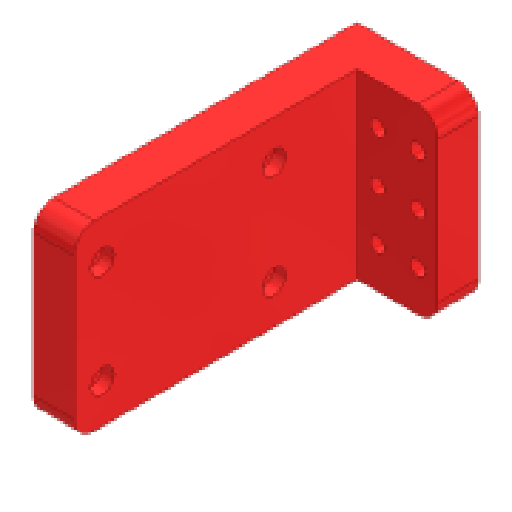
# Autodesk Inventor part: Uchwyt_konwerter
Saved by Autodesk Inventor 2024.3 (Build 283343000, 343)
## iProperties
Created: 2025-06-30
Part Number: Uchwyt_konwerter
Material: PET Plastic
Document SubType Name: Modeling
Designer: PM
Density: 1.541 g/cm^3
Appearance: Light Red
Author: PM
Autodesk Inventor part; units mm, degrees
ref_plane "YZ Plane" through (0, 0, 0) normal (1, 0, 0) x (0, 1, 0)
ref_plane "XZ Plane" through (0, 0, 0) normal (0, 1, 0) x (-1, 0, 0)
ref_plane "XY Plane" through (0, 0, 0) normal (0, 0, 1) x (1, 0, 0)
sketch "Sketch1" plane through (0, 0, 0) normal (0, 0, 1) x (1, 0, 0)
  line L0 (-10, -22.5) -> (10, -22.5)
  line L1 (10, -22.5) -> (10, 22.5)
  line L2 (10, 22.5) -> (-10, 22.5)
  line L3 (-10, 22.5) -> (-10, -22.5)
  line L4 (-10, -22.5) -> (10, 22.5) construction
  line L5 (10, -22.5) -> (-10, 22.5) construction
  line L6 (-10, 22.5) -> (-20, 22.5)
  line L7 (-20, 22.5) -> (-20, -22.5)
  line L8 (-20, -22.5) -> (-10, -22.5)
  line L9 (-10, -22.5) -> (-10, 22.5)
  point P0 (0, 0)
  dimension "d0" = 20
  dimension "d1" = 45
  dimension "d2" = 10
  constraints: 20 end point, 4 parallel, 2 horizontal, 2 midpoint, 2 perpendicular, 1 horizontal alignment
  measures "d0" distance of L1.end L2.end
  measures "d1" distance of L0.end L1.end
  measures "d2" distance of L2.end L6.end
extrude "Extrusion1" add sketch "Sketch1" along normal blind 10 contours L3 L2 L1 L0
sketch "Sketch2" plane through (0, 0, 10) normal (0, 0, 1) x (1, 0, 0)
  line L0 (5, -12.5) -> (-5, -12.5) construction
  line L1 (-5, -12.5) -> (-5, 12.5) construction
  line L2 (-5, 12.5) -> (5, 12.5) construction
  line L3 (5, 12.5) -> (5, -12.5) construction
  line L4 (5, -12.5) -> (-5, 12.5) construction
  line L5 (-5, -12.5) -> (5, 12.5) construction
  point P0 (0, 0)
  point P1 (-5, 0)
  point P2 (5, 0)
  dimension "d5" = 10
  dimension "d6" = 25
  constraints: 12 end point, 4 coincident, 4 midpoint, 2 parallel, 1 horizontal, 1 perpendicular
  measures "d5" distance of L1.end L2.end
  measures "d6" distance of L0.end L1.end
hole "Hole1" at (-5, 12.5, 10) at (5, 12.5, 10) at (5, -12.5, 10) at (-5, -12.5, 10) at (-5, 0, 10) at (5, 0, 10) direction (0, 0, -1) diameter 3.6 end through all clearance for "Countersunk Flat Head Screw DIN EN ISO 2009" size "M3" standard "DIN"
sketch "Sketch3" plane through (0, 0, 0) normal (0, 0, 1) x (1, 0, 0)
  line L0 (-10, 22.5) -> (-10, -22.5) projected
  line L1 (-10, 22.5) -> (-20, 22.5)
  line L2 (-20, 22.5) -> (-20, -22.5)
  line L3 (-20, -22.5) -> (-10, -22.5)
  line L4 (-10, -22.5) -> (-10, 22.5)
  point P0 (0, 0)
  dimension "d14" = 10
  constraints: 8 end point, 2 parallel, 1 horizontal, 1 horizontal alignment, 1 perpendicular
  measures "d14" distance of L0.start L1.end
extrude "Extrusion2" add sketch "Sketch3" along normal blind 80
sketch "Sketch4" plane through (-10, -22.5, 10) normal (1, 0, 0) x (0, 0, -1)
  line L0 (-63, 9.75) -> (-20.5, 9.75)
  line L1 (-20.5, 9.75) -> (-20.5, 35.25)
  line L2 (-20.5, 35.25) -> (-63, 35.25)
  line L3 (-63, 35.25) -> (-63, 9.75)
  line L4 (-63, 9.75) -> (-20.5, 35.25) construction
  line L5 (-20.5, 9.75) -> (-63, 35.25) construction
  line L6 (0, 0) -> (0, 45) projected
  line L7 (-70, 0) -> (-70, 45) projected
  line L8 (0, 45) -> (-70, 45) projected
  point P0 (10, 22.5)
  point P1 (-41.75, 22.5)
  point P2 (-70, 22.5)
  dimension "d17" = 42.5
  dimension "d18" = 25.5
  dimension "d19" = 7
  constraints: 12 end point, 4 coincident, 3 midpoint, 2 parallel, 1 horizontal, 1 horizontal alignment, 1 perpendicular
  measures "d17" distance of L2.end L1.end
  measures "d18" distance of L1.end L0.end
  measures "d19" distance between parallel lines of L7 L3
hole "Hole2" at (-10, 12.75, 73) at (-10, -12.75, 73) at (-10, 12.75, 30.5) at (-10, -12.75, 30.5) direction (-1, 0, 0) diameter 3 end through all clearance for "Countersunk Flat Head Screw DIN EN ISO 2009" size "M2.5" standard "DIN"
sketch "Sketch5" plane through (-10, -22.5, 10) normal (1, 0, 0) x (0, 0, -1)
  circle A0 centre (-63, 35.25) radius 1.5 projected
  circle A1 centre (-20.5, 35.25) radius 1.5 projected
  circle A2 centre (-20.5, 9.75) radius 1.5 projected
  circle A3 centre (-63, 9.75) radius 1.5 projected
  point P0 (10, 22.5)
hole "Hole3" at (-10, 12.75, 73) at (-10, 12.75, 30.5) at (-10, -12.75, 30.5) at (-10, -12.75, 73) direction (-1, 0, 0) diameter 5.8 depth 3
fillet "Fillet1" radius 5 4 edges at (-15, 22.5, 80) (-15, -22.5, 80) (10, 22.5, 5) (10, -22.5, 5)
body "Solid1"
